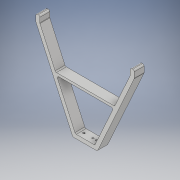
# Autodesk Inventor part: PatasColaTrasera
Saved by Autodesk Inventor 2019 (Build 230136000, 136)
## iProperties
Created: 2019-05-03
Part Number: PatasColaTrasera
Material: Generic
Document SubType Name: Modeling
Designer: Kenny
Density: 1 g/cm^3
Appearance: Default
Author: Kenny
Autodesk Inventor part; units mm, degrees
ref_plane "YZ Plane" through (0, 0, 0) normal (1, 0, 0) x (0, 1, 0)
ref_plane "XZ Plane" through (0, 0, 0) normal (0, 1, 0) x (-1, 0, 0)
ref_plane "XY Plane" through (0, 0, 0) normal (0, 0, 1) x (1, 0, 0)
sketch "Sketch2" plane through (0, 0, 0) normal (0, 0, 1) x (1, 0, 0)
  line L0 (0, 0) -> (200, 0) construction
  line L1 (200, 0) -> (200, 180) construction
  line L2 (200, 180) -> (0, 180) construction
  line L3 (0, 180) -> (0, 0) construction
  line L4 (0, 0) -> (75, 0) construction
  line L5 (75, 0) -> (125, 0)
  line L6 (125, 0) -> (200, 0) construction
  line L7 (0, 180) -> (0, 165)
  line L8 (200, 180) -> (200, 165)
  line L9 (200, 165) -> (125, 0)
  line L10 (75, 0) -> (0, 165)
  line L11 (0, 180) -> (8, 180)
  line L12 (200, 180) -> (192, 180)
  line L13 (119.8487, 8) -> (80.1513, 8)
  line L14 (8, 166.7329) -> (39.8628, 96.6347)
  line L15 (192, 166.7329) -> (160.1372, 96.6347)
  line L16 (160.1372, 96.6347) -> (39.8628, 96.6347)
  line L17 (8, 166.7329) -> (8, 180)
  line L18 (192, 166.7329) -> (192, 180)
  line L19 (42.1356, 91.6347) -> (80.1513, 8)
  line L20 (157.8644, 91.6347) -> (119.8487, 8)
  line L21 (42.1356, 91.6347) -> (157.8644, 91.6347)
  dimension "d0" = 200
  dimension "d1" = 180
  dimension "d2" = 75
  dimension "d3" = 50
  dimension "d4" = 15
  dimension "d5" = 15
  dimension "d6" = 8
  dimension "d7" = 8
  dimension "d10" = 77
  dimension "d11" = 8
  dimension "d12" = 8
  dimension "d14" = 8
  dimension "d15" = 5
  constraints: 44 end point, 9 parallel, 6 point on line, 3 horizontal, 1 collinear, 1 perpendicular
  measures "d0" distance of L2.end L1.end
  measures "d1" distance of L1.end L0.end
  measures "d2" distance of L0.start L4.end
  measures "d3" distance of L4.end L5.end
  measures "d4" distance of L2.end L7.end
  measures "d5" distance of L1.end L8.end
  measures "d6" distance of L2.end L11.end
  measures "d7" distance of L1.end L12.end
  measures "d10" distance of L14.start L14.end
  measures "d11" distance between parallel lines of L10 L14
  measures "d12" distance between parallel lines of L9 L15
  measures "d14" distance between parallel lines of L0 L13
  measures "d15" distance between parallel lines of L21 L16
extrude "Extrusion1" add sketch "Sketch2" along normal blind 20
fillet "Fillet1" radius 3 16 edges at (8, 180, 10) (0, 180, 10) (8, 166.7329, 10) (0, 165, 10) (200, 180, 10) (192, 180, 10) (200, 165, 10) (192, 166.7329, 10) (39.8628, 96.6347, 10) (42.1356, 91.6347, 10) (160.1372, 96.6347, 10) (157.8644, 91.6347, 10) (80.1513, 8, 10) (119.8487, 8, 10) (125, 0, 10) (75, 0, 10)
sketch "Sketch5" plane through (46.7946, 91.6347, 20) normal (0, -1, 0) x (1, 0, 0)
  line L0 (106.4109, -20) -> (0, -20) projected
  line L1 (0, -20) -> (0, 0) projected
  point P0 (-46.7946, -20)
  point P1 (40.2055, -10)
  point P2 (41.2055, -10)
  point P3 (59.2055, -10)
  point P4 (66.2055, -10)
  dimension "d39" = 1
  dimension "d40" = 18
  dimension "d41" = 7
  dimension "d42" = 10
  dimension "d43" = 40.2055
  constraints: 3 horizontal alignment
  measures "d39" distance of point (41.206, -10) point (40.206, -10)
  measures "d40" distance of point (59.205, -10) point (41.206, -10)
  measures "d41" distance of point (66.206, -10) point (59.205, -10)
  measures "d42" distance from line of L0 point (40.206, -10)
  measures "d43" distance from line of L1 point (40.206, -10)
hole "Hole1" at (87.0001, 91.6347, 10) at (88.0001, 91.6347, 10) at (106.0001, 91.6347, 10) at (113.0001, 91.6347, 10) direction (0, -1, 0) diameter 3.5 end through all
sketch "Sketch6" plane through (76.9317, 0, 0) normal (0, -1, 0) x (1, 0, 0)
  arc A0 (10.5683, 11.6771) -> (10.5683, 8.3229) centre (10.0683, 10) ccw projected
  line L0 (10.0683, 11.75) -> (11.0683, 11.75)
  line L1 (10.0683, 8.25) -> (11.0683, 8.25)
  arc A1 (10.5683, 8.3229) -> (10.5683, 11.6771) centre (11.0683, 10) ccw projected
  point P0 (-76.9317, 0)
  constraints: 4 end point, 4 point on circle, 4 tangent, 2 horizontal
extrude "Extrusion2" cut sketch "Sketch6" against normal blind 8 contours A0 L0 A1 | A0 A1 L1
body "Solid1"
